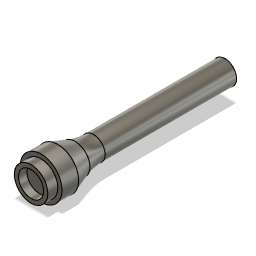
Axial+rotator+(right) (Autodesk Fusion 360 design; units mm, degrees)
Autodesk Fusion 360 part; units mm, degrees
sketch "Sketch5" plane through (0, 0, 0) normal (0, 0, 1) x (1, 0, 0)
  circle A0 centre (0, 0) radius 12.5
  circle A1 centre (0, 0) radius 10
  circle A2 centre (0, 0) radius 7.5
  dimension "d32" = 25
  dimension "d33" = 20
  dimension "d34" = 15
  constraint coincident A0.centre A1.centre
  constraint concentric A1 A2
  measures "d32" diameter of A0
  measures "d33" diameter of A1
  measures "d34" diameter of A2
extrude "Extrude8" add sketch "Sketch5" along normal blind 10 contours A0
extrude "Extrude9" add sketch "Sketch5" along normal blind 16 contours A1
sketch "Sketch6" plane through (0, 0, 0) normal (1, 0, 0) x (0, 0, -1)
  line L0 (0, 0) -> (100, 0)
  line L1 (100, 0) -> (100, 7)
  line L2 (0, 12.5) -> (0, -12.5)
  line L3 (100, 7) -> (21.3505, 7)
  line L4 (0, 12.5) -> (10.3963, 8.8615)
  arc A0 (10.3963, 8.8615) -> (21.3505, 7) centre (21.3505, 40.1609) ccw
  dimension "d39" = 100
  dimension "d40" = 7
  dimension "d43" = 33.1609
  constraint coincident L0.start origin
  constraint horizontal L0
  constraint perpendicular L0 L1
  constraint perpendicular L2 L3
  constraint coincident L2.start L4.start
  constraint tangent L4 A0
  constraint tangent L3 A0
  measures "d39" distance of L0.start L0.end
  measures "d40" distance of L0.end L1.end
  measures "d43" radius of A0
revolve "Revolve2" add sketch "Sketch6" angle 360 about axis through (0, 0, 0) along (0, 0, -1)
sketch "Sketch7" plane through (0, 0, -100) normal (0, 0, -1) x (-1, 0, 0)
  circle A0 centre (0, 0) radius 7
  line L0 (-1.5, 2) -> (1.5, 2)
  arc A1 (-1.5, 2) -> (1.5, 2) centre (0, 0) ccw
  dimension "d1" = 5
  measures "d1" diameter of A1
extrude "Extrude10" cut sketch "Sketch7" against normal blind 15 contours L0 A1
extrude "Extrude11" add 1 faces at (-1.613, 0.9883, 0) along direction (0, 0, 1) blind 11
